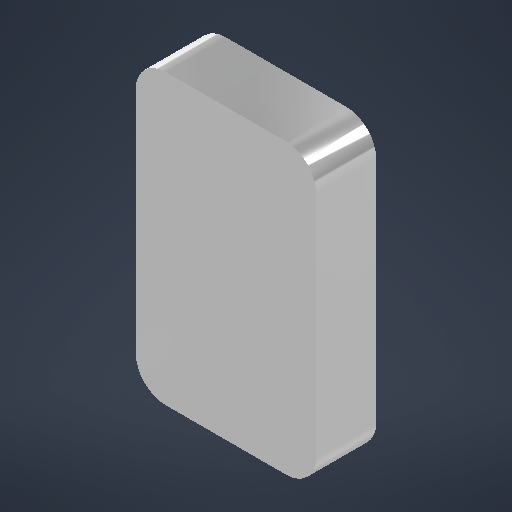
# Autodesk Inventor part: Backplate
Saved by Autodesk Inventor 2025.1 (Build 291241020, 241B)
## iProperties
Created: 2024-10-06
Part Number: Backplate
Material: Aluminum 6061
Document SubType Name: Modeling
Designer: Sora
Density: 2.7 g/cm^3
Appearance: Aluminum - Flat
Author: Sora
Autodesk Inventor part; units mm, degrees
ref_plane "YZ Plane" through (0, 0, 0) normal (1, 0, 0) x (0, 1, 0)
ref_plane "XZ Plane" through (0, 0, 0) normal (0, 1, 0) x (-1, 0, 0)
ref_plane "XY Plane" through (0, 0, 0) normal (0, 0, 1) x (1, 0, 0)
sketch "Sketch1" plane through (0, 0, 0) normal (0, 0, 1) x (1, 0, 0)
  line L0 (-15, 19) -> (-15, -19) projected
  arc A0 (-10, 24) -> (-15, 19) centre (-10, 19) ccw projected
  line L1 (10, 24) -> (-10, 24) projected
  arc A1 (15, 19) -> (10, 24) centre (10, 19) ccw projected
  line L2 (15, -19) -> (15, 19) projected
  arc A2 (10, -24) -> (15, -19) centre (10, -19) ccw projected
  line L3 (-10, -24) -> (10, -24) projected
  arc A3 (-15, -19) -> (-10, -24) centre (-10, -19) ccw projected
  point P0 (0, 0)
extrude "Extrusion1" add sketch "Sketch1" along normal blind 10
sketch "Sketch2" plane through (0, 0, 0) normal (0, 0, -1) x (-1, 0, 0)
  circle A0 centre (-10, 19) radius 1.6 projected
  circle A1 centre (-10, -19) radius 1.6 projected
  arc A2 (10, -24) -> (15, -19) centre (10, -19) ccw projected
  line L0 (15, 19) -> (15, -19) projected
  arc A3 (15, 19) -> (10, 24) centre (10, 19) ccw projected
  line L1 (-10, 24) -> (10, 24) projected
  arc A4 (-10, 24) -> (-15, 19) centre (-10, 19) ccw projected
  line L2 (-15, -19) -> (-15, 19) projected
  arc A5 (-15, -19) -> (-10, -24) centre (-10, -19) ccw projected
  line L3 (10, -24) -> (-10, -24) projected
  circle A6 centre (10, -19) radius 1.6 projected
  circle A7 centre (10, 19) radius 1.6 projected
hole "Hole1" at (10, 19, 0) at (10, -19, 0) at (-10, -19, 0) at (-10, 19, 0) direction (0, 0, 1) diameter 2.459 depth 8 tip angle 118 thread size "M3x0.5" class "6H" standard "ANSI Metric M Profile"
sketch "Sketch3" plane through (0, 0, 0) normal (0, 0, -1) x (-1, 0, 0)
  circle A0 centre (10, 19) radius 1.2295 construction
  circle A1 centre (10, -19) radius 1.2295 construction
  circle A2 centre (-10, -19) radius 1.2295 construction
  circle A3 centre (-10, 19) radius 1.2295 construction
  arc A4 (10, -24) -> (15, -19) centre (10, -19) ccw projected
  line L0 (15, 19) -> (15, -19) projected
  arc A5 (15, 19) -> (10, 24) centre (10, 19) ccw projected
  line L1 (-10, 24) -> (10, 24) projected
  arc A6 (-10, 24) -> (-15, 19) centre (-10, 19) ccw projected
  line L2 (-15, -19) -> (-15, 19) projected
  arc A7 (-15, -19) -> (-10, -24) centre (-10, -19) ccw projected
  line L3 (10, -24) -> (-10, -24) projected
  arc A8 (15, 19) -> (10, 24) centre (10, 19) ccw projected
  line L4 (-10, 24) -> (10, 24) projected
  arc A9 (-10, 24) -> (-15, 19) centre (-10, 19) ccw projected
  line L5 (-15, -19) -> (-15, 19) projected
  arc A10 (-15, -19) -> (-10, -24) centre (-10, -19) ccw projected
  line L6 (10, -24) -> (-10, -24) projected
  arc A11 (10, -24) -> (15, -19) centre (10, -19) ccw projected
  line L7 (15, 19) -> (15, -19) projected
  circle A12 centre (11.6971, -20.6971) radius 0.25 construction
  circle A13 centre (12.4, -19) radius 0.25 construction
  circle A14 centre (10, -21.4) radius 0.25 construction
  circle A15 centre (10, -19) radius 1.6 construction
  circle A16 centre (11.6971, -17.3029) radius 0.25 construction
  circle A17 centre (10, -16.6) radius 0.25 construction
  circle A18 centre (8.3029, -20.6971) radius 0.25 construction
  circle A19 centre (7.6, -19) radius 0.25 construction
  circle A20 centre (8.3029, -17.3029) radius 0.25 construction
  circle A21 centre (2.62, -11.54) radius 0.5 construction
  circle A22 centre (0.08, -11.54) radius 0.5 construction
  circle A23 centre (11.3, -10.4) radius 0.4953 construction
  circle A24 centre (12.316, -5.32) radius 0.4953 construction
  circle A25 centre (10.284, -5.32) radius 0.4953 construction
  circle A26 centre (2.62, -9) radius 0.5 construction
  circle A27 centre (0.08, -9) radius 0.5 construction
  circle A28 centre (-2.46, -11.54) radius 0.5 construction
  circle A29 centre (-8.3029, -20.6971) radius 0.25 construction
  circle A30 centre (-7.6, -19) radius 0.25 construction
  circle A31 centre (-10, -21.4) radius 0.25 construction
  circle A32 centre (-10, -19) radius 1.6 construction
  circle A33 centre (-8.3029, -17.3029) radius 0.25 construction
  circle A34 centre (-10, -16.6) radius 0.25 construction
  circle A35 centre (-11.6971, -20.6971) radius 0.25 construction
  circle A36 centre (-12.4, -19) radius 0.25 construction
  circle A37 centre (-11.6971, -17.3029) radius 0.25 construction
  circle A38 centre (-2.46, -9) radius 0.5 construction
  circle A39 centre (-13.3, -3.2) radius 0.45 construction
  circle A40 centre (-13.3, -0.2) radius 0.45 construction
  circle A41 centre (10.7, 8.9) radius 0.1 construction
  circle A42 centre (9.85, 8.9) radius 0.1 construction
  circle A43 centre (10.7, 9.7) radius 0.1 construction
  circle A44 centre (9.85, 9.7) radius 0.1 construction
  circle A45 centre (9, 8.9) radius 0.1 construction
  circle A46 centre (9, 9.7) radius 0.1 construction
  circle A47 centre (11.6971, 17.3029) radius 0.25 construction
  circle A48 centre (12.4, 19) radius 0.25 construction
  circle A49 centre (10, 16.6) radius 0.25 construction
  circle A50 centre (10, 19) radius 1.6 construction
  circle A51 centre (11.6971, 20.6971) radius 0.25 construction
  circle A52 centre (10, 21.4) radius 0.25 construction
  circle A53 centre (8.3029, 17.3029) radius 0.25 construction
  circle A54 centre (7.6, 19) radius 0.25 construction
  circle A55 centre (8.3029, 20.6971) radius 0.25 construction
  arc A56 (4.02, 16.62) -> (4.62, 16.62) centre (4.32, 16.62) ccw construction
  line L8 (4.02, 17.72) -> (4.02, 16.62) construction
  arc A57 (4.62, 17.72) -> (4.02, 17.72) centre (4.32, 17.72) ccw construction
  line L9 (4.62, 16.62) -> (4.62, 17.72) construction
  circle A58 centre (2.89, 17.7) radius 0.325 construction
  arc A59 (4.02, 21.05) -> (4.62, 21.05) centre (4.32, 21.05) ccw construction
  line L10 (4.02, 21.65) -> (4.02, 21.05) construction
  arc A60 (4.62, 21.65) -> (4.02, 21.65) centre (4.32, 21.65) ccw construction
  line L11 (4.62, 21.05) -> (4.62, 21.65) construction
  circle A61 centre (-2.89, 17.7) radius 0.325 construction
  arc A62 (-4.62, 16.62) -> (-4.02, 16.62) centre (-4.32, 16.62) ccw construction
  line L12 (-4.62, 17.72) -> (-4.62, 16.62) construction
  arc A63 (-4.02, 17.72) -> (-4.62, 17.72) centre (-4.32, 17.72) ccw construction
  line L13 (-4.02, 16.62) -> (-4.02, 17.72) construction
  arc A64 (-4.62, 21.05) -> (-4.02, 21.05) centre (-4.32, 21.05) ccw construction
  line L14 (-4.62, 21.65) -> (-4.62, 21.05) construction
  arc A65 (-4.02, 21.65) -> (-4.62, 21.65) centre (-4.32, 21.65) ccw construction
  line L15 (-4.02, 21.05) -> (-4.02, 21.65) construction
  circle A66 centre (-8.3029, 17.3029) radius 0.25 construction
  circle A67 centre (-7.6, 19) radius 0.25 construction
  circle A68 centre (-10, 16.6) radius 0.25 construction
  circle A69 centre (-10, 19) radius 1.6 construction
  circle A70 centre (-8.3029, 20.6971) radius 0.25 construction
  circle A71 centre (-10, 21.4) radius 0.25 construction
  circle A72 centre (-11.6971, 17.3029) radius 0.25 construction
  circle A73 centre (-12.4, 19) radius 0.25 construction
  circle A74 centre (-11.6971, 20.6971) radius 0.25 construction
  line L16 (11.3, -10.4) -> (11.3, -5.32) construction
  line L17 (13.8, -10.4) -> (13.8, -5.32)
  line L18 (8.8, -5.32) -> (8.8, -10.4)
  arc A75 (8.8, -10.4) -> (13.8, -10.4) centre (11.3, -10.4) ccw
  arc A76 (13.8, -5.32) -> (8.8, -5.32) centre (11.3, -5.32) ccw
  line L19 (11.3, -5.32) -> (12.316, -5.32) construction
  line L20 (-4.32, 17.72) -> (4.32, 17.72) construction
  line L21 (4.32, 21.05) -> (-4.32, 21.05) construction
  line L22 (0, 17.72) -> (0, 21.05) construction
  line L23 (-4, 19.385) -> (4, 19.385) construction
  line L24 (-4, 15.885) -> (4, 15.885)
  line L25 (4, 22.885) -> (-4, 22.885)
  arc A77 (-4, 22.885) -> (-4, 15.885) centre (-4, 19.385) ccw
  arc A78 (4, 15.885) -> (4, 22.885) centre (4, 19.385) ccw
  line L26 (-2.46, -11.54) -> (2.62, -9) construction
  line L27 (2.62, -11.54) -> (-2.46, -9) construction
  line L28 (-2.92, -10.27) -> (3.08, -10.27) construction
  line L29 (-2.92, -14.27) -> (3.08, -14.27)
  line L30 (3.08, -6.27) -> (-2.92, -6.27)
  arc A79 (-2.92, -6.27) -> (-2.92, -14.27) centre (-2.92, -10.27) ccw
  arc A80 (3.08, -14.27) -> (3.08, -6.27) centre (3.08, -10.27) ccw
  point P0 (0, 0)
  point P1 (11.3, -7.86)
  point P2 (0, 19.385)
  point P3 (0.08, -10.27)
  dimension "d10" = 5
  dimension "d16" = 4
  dimension "d17" = 7
  dimension "d18" = 3
  dimension "d19" = 8
  constraints: 36 end point, 12 point on circle, 12 tangent, 7 midpoint, 6 centre point, 5 horizontal, 3 parallel, 1 vertical
  measures "d10" diameter of A76
  measures "d16" distance of point (0, 19.385) L23.end
  measures "d17" diameter of A78
  measures "d18" distance of point (0.08, -10.27) L28.end
  measures "d19" diameter of A80
extrude "Extrusion2" cut sketch "Sketch3" against normal blind 5 contours A75 L18 A76 L17 | A77 L25 A78 L24 | A79 L30 A80 L29
body "Solid1"
